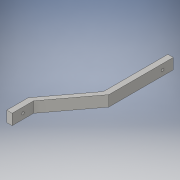
# Autodesk Inventor part: arm2
Saved by Autodesk Inventor 2016 (Build 200138000, 138)
## iProperties
Created: 2016-01-18
Part Number: arm2
Material: Generic
Document SubType Name: Modeling
Designer: Thariq
Density: 1 g/cm^3
Appearance: Default
Author: Thariq
Autodesk Inventor part; units mm, degrees
ref_plane "YZ Plane" through (0, 0, 0) normal (1, 0, 0) x (0, 1, 0)
ref_plane "XZ Plane" through (0, 0, 0) normal (0, 1, 0) x (-1, 0, 0)
ref_plane "XY Plane" through (0, 0, 0) normal (0, 0, 1) x (1, 0, 0)
sketch "Sketch1" plane through (0, 0, 0) normal (0, 1, 0) x (-1, 0, 0)
  line L0 (127, 143.8324) -> (0, 143.8324)
  line L1 (0, 143.8324) -> (0, -160.9676)
  line L2 (0, -160.9676) -> (127, -160.9676)
  line L3 (127, -160.9676) -> (127, 143.8324)
  line L4 (0, -160.9676) -> (12.7, -160.9676)
  line L5 (12.7, -160.9676) -> (12.7, -8.5676)
  line L6 (12.7, -8.5676) -> (0, -8.5676)
  line L7 (0, -8.5676) -> (0, -160.9676)
  line L8 (12.7, -8.5676) -> (88.9, 93.0324)
  line L9 (0, -8.5676) -> (76.2, 93.0324)
  line L10 (127, 143.8324) -> (76.2, 143.8324)
  line L11 (76.2, 143.8324) -> (76.2, 93.0324)
  line L12 (88.9, 93.0324) -> (127, 93.0324)
  line L13 (127, 93.0324) -> (127, 143.8324)
  line L14 (88.9, 93.0324) -> (88.9, 143.8324)
  point P0 (0, 0)
  point P1 (114.3, 143.8324)
  dimension "d0" = 304.8
  dimension "d1" = 127
  dimension "d2" = 12.7
  dimension "d3" = 152.4
  dimension "d16" = 50.8
  dimension "d17" = 0
  dimension "d18" = 12.7
  constraints: 30 end point, 7 parallel, 4 perpendicular, 3 horizontal, 3 point on line
  measures "d0" distance between parallel lines of L2 L0
  measures "d1" distance between parallel lines of L3 L1
  measures "d2" distance between parallel lines of L1 L5
  measures "d3" distance between parallel lines of L6 L2
  measures "d16" distance between parallel lines of L10 L12
  measures "d17" distance between parallel lines of L10 L0
  measures "d18" distance between parallel lines of L14 L11
extrude "Extrusion1" add sketch "Sketch1" along normal blind 25.4 contours L14 L8 L6 L9 L11 L0 | L5 L2 L1 L6
sketch "Sketch2" plane through (0, 0, -8.5676) normal (1, 0, 0) x (0, 0, -1)
  circle A0 centre (127, 12.7) radius 3.175
  line L0 (0, 0) -> (152.4, 0) projected
  line L1 (152.4, 0) -> (152.4, 25.4) projected
  point P0 (-8.5676, 0)
  dimension "d6" = 6.35
  dimension "d7" = 12.7
  dimension "d8" = 25.4
  constraints: 1 centre point
  measures "d6" diameter of A0
  measures "d7" distance from line of L0 A0.centre
  measures "d8" distance from line of A0.centre L1
extrude "Extrusion2" cut sketch "Sketch2" against normal through all
sketch "Sketch4" plane through (-76.2, 0, 143.8324) normal (1, 0, 0) x (0, 0, -1)
  circle A0 centre (25.4, 12.7) radius 3.175
  line L0 (0, 0) -> (50.8, 0) projected
  line L1 (0, 0) -> (0, 25.4) projected
  point P0 (143.8324, 0)
  dimension "d19" = 6.35
  dimension "d20" = 12.7
  dimension "d21" = 25.4
  constraints: 1 centre point
  measures "d19" diameter of A0
  measures "d20" distance from line of L0 A0.centre
  measures "d21" distance from line of L1 A0.centre
extrude "Extrusion4" cut sketch "Sketch4" against normal through all
body "Solid1"
